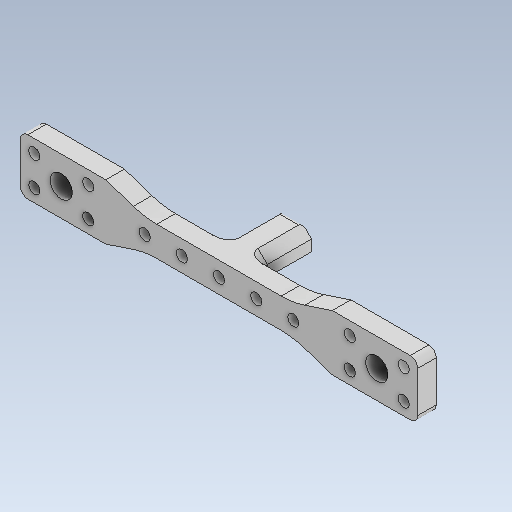
# Autodesk Inventor part: carbon_fiber_fixer_1
Saved by Autodesk Inventor 2020 (Build 240168000, 168)
## iProperties
Created: 2019-09-06
Part Number: carbon_fiber_fixer_1
Material: Generic
Document SubType Name: Modeling
Designer: psrob
Density: 1 g/cm^3
Appearance: Default
Author: psrob
Autodesk Inventor part; units mm, degrees
ref_plane "YZ Plane" through (0, 0, 0) normal (1, 0, 0) x (0, 1, 0)
ref_plane "XZ Plane" through (0, 0, 0) normal (0, 1, 0) x (-1, 0, 0)
ref_plane "XY Plane" through (0, 0, 0) normal (0, 0, 1) x (1, 0, 0)
sketch "Sketch1" plane through (0, 0, 0) normal (0, 0, 1) x (1, 0, 0)
  circle A0 centre (-100.25, -3.5) radius 1.5 projected
  circle A1 centre (-100.25, -11.5) radius 1.5 projected
  line L0 (-104, 0) -> (-96.5, 0) projected
  line L1 (-104, 0) -> (-104, -15) projected
  line L2 (-96.5, -15) -> (-104, -15) projected
  line L3 (-96.5, 0) -> (-96.5, -15) projected
  circle A2 centre (-85.75, -3.5) radius 1.5 projected
  circle A3 centre (-85.75, -11.5) radius 1.5 projected
  line L4 (-90.5, 0) -> (-81, 0) projected
  line L5 (-90.5, 0) -> (-90.5, -15) projected
  line L6 (-81, -15) -> (-90.5, -15) projected
  line L7 (-81, 0) -> (-81, -15) projected
  circle A4 centre (-15.25, -11.5) radius 1.5 projected
  circle A5 centre (-15.25, -3.5) radius 1.5 projected
  line L8 (-20, 0) -> (-10.5, 0) projected
  line L9 (-20, 0) -> (-20, -15) projected
  line L10 (-10.5, -15) -> (-20, -15) projected
  line L11 (-10.5, 0) -> (-10.5, -15) projected
  circle A6 centre (-0.75, -3.5) radius 1.5 projected
  circle A7 centre (-0.75, -11.5) radius 1.5 projected
  line L12 (-4.5, 0) -> (3, 0) projected
  line L13 (-4.5, 0) -> (-4.5, -15) projected
  line L14 (3, -15) -> (-4.5, -15) projected
  line L15 (3, 0) -> (3, -15) projected
  line L16 (-104, -15) -> (3, -15)
  line L17 (3, -15) -> (3, 0)
  line L18 (3, 0) -> (-104, 0)
  line L19 (-104, 0) -> (-104, -15)
  line L20 (-50.5, -15) -> (-50.5, 0)
  line L21 (-70.5, -11.5) -> (-70.5, -3.5)
  line L22 (-70.5, -3.5) -> (-30.5, -3.5)
  line L23 (-30.5, -3.5) -> (-30.5, -11.5)
  line L24 (-30.5, -11.5) -> (-70.5, -11.5)
  line L25 (-70.5, -11.5) -> (-30.5, -3.5) construction
  line L26 (-70.5, -3.5) -> (-30.5, -11.5) construction
  line L27 (-70.5, -3.5) -> (-81, 0)
  line L28 (-30.5, -3.5) -> (-20, 0)
  line L29 (-30.5, -11.5) -> (-20, -15)
  line L30 (-70.5, -11.5) -> (-81, -15)
  point P0 (0, 0)
  point P1 (-50.5, -7.5)
  dimension "d0" = 8
  dimension "d1" = 40
  constraints: 30 end point, 6 parallel, 5 midpoint, 2 perpendicular, 1 horizontal
  measures "d0" distance of L21.start L21.end
  measures "d1" distance of L21.end L22.end
extrude "Extrusion1" add sketch "Sketch1" along normal blind 5 contours L0 L3 L2 L1 | L18 L5 L16 L3 | L4 L7 L6 L5 | L27 L21 L30 L7 | L22 L20 L24 L21 | L8 L11 L10 L9 | L9 L29 L23 L28 | L22 L23 L24 L20 | L18 L13 L16 L11 | L12 L15 L14 L13
sketch "Sketch2" plane through (0, 0, 5) normal (0, 0, 1) x (1, 0, 0)
  line L0 (-81, 0) -> (-104, 0) projected
  line L1 (-104, 0) -> (-104, -15) projected
  line L2 (-104, -15) -> (-81, -15) projected
  line L3 (-81, -15) -> (-70.5, -11.5) projected
  line L4 (-70.5, -11.5) -> (-30.5, -11.5) projected
  line L5 (-30.5, -11.5) -> (-20, -15) projected
  line L6 (-20, -15) -> (3, -15) projected
  line L7 (3, -15) -> (3, 0) projected
  line L8 (3, 0) -> (-20, 0) projected
  line L9 (-20, 0) -> (-30.5, -3.5) projected
  line L10 (-30.5, -3.5) -> (-70.5, -3.5) projected
  line L11 (-70.5, -3.5) -> (-81, 0) projected
  circle A0 centre (-100.25, -3.5) radius 1.5 projected
  circle A1 centre (-100.25, -11.5) radius 1.5 projected
  circle A2 centre (-85.75, -3.5) radius 1.5 projected
  circle A3 centre (-85.75, -11.5) radius 1.5 projected
  circle A4 centre (-15.25, -11.5) radius 1.5 projected
  circle A5 centre (-15.25, -3.5) radius 1.5 projected
  circle A6 centre (-0.75, -3.5) radius 1.5 projected
  circle A7 centre (-0.75, -11.5) radius 1.5 projected
  line L12 (-70.5, -11.5) -> (-30.5, -11.5) projected
  line L13 (-50.5, -11.5) -> (-50.5, -3.5)
  line L14 (-30.5, -3.5) -> (-70.5, -3.5) projected
  line L15 (-50.5, -7.5) -> (-60.5, -7.5)
  line L16 (-60.5, -7.5) -> (-70.5, -7.5)
  line L17 (-50.5, -7.5) -> (-40.5, -7.5)
  line L18 (-40.5, -7.5) -> (-30.5, -7.5)
  circle A8 centre (-70.5, -7.5) radius 1.5
  circle A9 centre (-60.5, -7.5) radius 1.5
  circle A10 centre (-50.5, -7.5) radius 1.5
  circle A11 centre (-40.5, -7.5) radius 1.5
  circle A12 centre (-30.5, -7.5) radius 1.5
  point P0 (0, 0)
  dimension "d4" = 10
  dimension "d5" = 10
  dimension "d6" = 10
  dimension "d7" = 10
  dimension "d8" = 3
  dimension "d9" = 3
  dimension "d10" = 3
  dimension "d11" = 3
  dimension "d12" = 3
  constraints: 10 end point, 5 centre point, 5 coincident, 3 midpoint, 2 horizontal, 1 parallel, 1 point on line
  measures "d4" distance of L15.start L15.end
  measures "d5" distance of L15.end L16.end
  measures "d6" distance of L15.start L17.end
  measures "d7" distance of L17.end L18.end
  measures "d8" diameter of A8
  measures "d9" diameter of A9
  measures "d10" diameter of A10
  measures "d11" diameter of A11
  measures "d12" diameter of A12
extrude "Extrusion2" cut sketch "Sketch2" against normal blind 5 contours A10 L17 L13 | L13 L15 A10 | L17 A10 L13 | L13 A10 L15 | A9 L16 L15 | L15 L16 A9 | A11 L18 L17 | L17 L18 A11 | A8 | A12
fillet "Fillet1" radius 2 4 edges at (-104, 0, 2.5) (-104, -15, 2.5) (3, -15, 2.5) (3, 0, 2.5)
sketch "Sketch3" plane through (0, 0, 5) normal (0, 0, 1) x (1, 0, 0)
  arc A0 (3, -2) -> (1, 0) centre (1, -2) ccw projected
  line L0 (1, 0) -> (-20, 0) projected
  line L1 (-20, 0) -> (-30.5, -3.5) projected
  line L2 (-30.5, -3.5) -> (-70.5, -3.5) projected
  line L3 (-70.5, -3.5) -> (-81, 0) projected
  line L4 (-81, 0) -> (-102, 0) projected
  arc A1 (-102, 0) -> (-104, -2) centre (-102, -2) ccw projected
  line L5 (-104, -2) -> (-104, -13) projected
  arc A2 (-104, -13) -> (-102, -15) centre (-102, -13) ccw projected
  line L6 (-102, -15) -> (-81, -15) projected
  line L7 (-81, -15) -> (-70.5, -11.5) projected
  line L8 (-70.5, -11.5) -> (-30.5, -11.5) projected
  line L9 (-30.5, -11.5) -> (-20, -15) projected
  line L10 (-20, -15) -> (1, -15) projected
  arc A3 (1, -15) -> (3, -13) centre (1, -13) ccw projected
  line L11 (3, -13) -> (3, -2) projected
  circle A4 centre (-50.5, -7.5) radius 1.5 projected
  circle A5 centre (-40.5, -7.5) radius 1.5 projected
  circle A6 centre (-60.5, -7.5) radius 1.5 projected
  circle A7 centre (-30.5, -7.5) radius 1.5 projected
  circle A8 centre (-70.5, -7.5) radius 1.5 projected
  circle A9 centre (-100.25, -3.5) radius 1.5 projected
  circle A10 centre (-100.25, -11.5) radius 1.5 projected
  circle A11 centre (-85.75, -3.5) radius 1.5 projected
  circle A12 centre (-85.75, -11.5) radius 1.5 projected
  circle A13 centre (-15.25, -11.5) radius 1.5 projected
  circle A14 centre (-15.25, -3.5) radius 1.5 projected
  circle A15 centre (-0.75, -3.5) radius 1.5 projected
  circle A16 centre (-0.75, -11.5) radius 1.5 projected
  line L12 (-55.5, -11.5) -> (-55.5, -3.5)
  line L13 (-55.5, -3.5) -> (-45.5, -3.5)
  line L14 (-45.5, -3.5) -> (-45.5, -11.5)
  line L15 (-45.5, -11.5) -> (-55.5, -11.5)
  circle A17 centre (-50.5, -7.5) radius 1.5 projected
  line L16 (-55.5, -11.5) -> (-45.5, -3.5) construction
  line L17 (-55.5, -3.5) -> (-45.5, -11.5) construction
  point P0 (0, 0)
  dimension "d16" = 8
  dimension "d17" = 10
  constraints: 12 end point, 2 midpoint, 2 parallel, 1 perpendicular
  measures "d16" distance of L12.start L12.end
  measures "d17" distance of L12.end L13.end
ref_plane "Work Plane1" through (-77, -15, -14.9044) normal (0, 0, 1) x (1, 0, 0)
extrude "Extrusion3" add sketch "Sketch3" against normal up to surface (19.9044 mm away) contours L14 L8 L12 L2
chamfer "Chamfer1" distance 2.5 angle 45 4 edges at (-45.5, -3.5, -7.4522) (-55.5, -3.5, -7.4522) (-45.5, -11.5, -7.4522) (-55.5, -11.5, -7.4522)
fillet "Fillet2" radius 3 6 edges at (-54.25, -10.25, 0) (-55.5, -7.5, 0) (-54.25, -4.75, 0) (-46.75, -10.25, 0) (-45.5, -7.5, 0) (-46.75, -4.75, 0)
fillet "Fillet3" radius 1 1 edges at (-50.5, -3.5, -14.9044)
fillet "Fillet4" radius 20 4 edges at (-70.5, -3.5, 2.5) (-30.5, -3.5, 2.5) (-70.5, -11.5, 2.5) (-30.5, -11.5, 2.5)
sketch "Sketch4" plane through (0, 0, 5) normal (0, 0, 1) x (1, 0, 0)
  circle A0 centre (-0.75, -11.5) radius 1.5 projected
  circle A1 centre (-0.75, -3.5) radius 1.5 projected
  circle A2 centre (-15.25, -3.5) radius 1.5 projected
  circle A3 centre (-15.25, -11.5) radius 1.5 projected
  circle A4 centre (-30.5, -7.5) radius 1.5 projected
  circle A5 centre (-40.5, -7.5) radius 1.5 projected
  circle A6 centre (-50.5, -7.5) radius 1.5 projected
  line L0 (-33.7456, -3.5) -> (-67.2544, -3.5) projected
  arc A7 (-73.579, -2.4737) -> (-67.2544, -3.5) centre (-67.2544, 16.5) ccw projected
  line L1 (-73.579, -2.4737) -> (-81, 0) projected
  line L2 (-81, 0) -> (-102, 0) projected
  arc A8 (-102, 0) -> (-104, -2) centre (-102, -2) ccw projected
  line L3 (-104, -2) -> (-104, -13) projected
  arc A9 (-104, -13) -> (-102, -15) centre (-102, -13) ccw projected
  line L4 (-102, -15) -> (-81, -15) projected
  line L5 (-81, -15) -> (-73.579, -12.5263) projected
  arc A10 (-67.2544, -11.5) -> (-73.579, -12.5263) centre (-67.2544, -31.5) ccw projected
  line L6 (-67.2544, -11.5) -> (-33.7456, -11.5) projected
  arc A11 (-27.421, -12.5263) -> (-33.7456, -11.5) centre (-33.7456, -31.5) ccw projected
  line L7 (-27.421, -12.5263) -> (-20, -15) projected
  line L8 (-20, -15) -> (1, -15) projected
  arc A12 (1, -15) -> (3, -13) centre (1, -13) ccw projected
  line L9 (3, -13) -> (3, -2) projected
  arc A13 (3, -2) -> (1, 0) centre (1, -2) ccw projected
  line L10 (1, 0) -> (-20, 0) projected
  line L11 (-20, 0) -> (-27.421, -2.4737) projected
  arc A14 (-33.7456, -3.5) -> (-27.421, -2.4737) centre (-33.7456, 16.5) ccw projected
  circle A15 centre (-60.5, -7.5) radius 1.5 projected
  circle A16 centre (-70.5, -7.5) radius 1.5 projected
  circle A17 centre (-100.25, -3.5) radius 1.5 projected
  circle A18 centre (-100.25, -11.5) radius 1.5 projected
  circle A19 centre (-85.75, -3.5) radius 1.5 projected
  circle A20 centre (-85.75, -11.5) radius 1.5 projected
  line L12 (-100.25, -3.5) -> (-85.75, -11.5)
  circle A21 centre (-85.75, -3.5) radius 1.5 projected
  line L13 (-85.75, -11.5) -> (-85.75, -3.5)
  circle A22 centre (-100.25, -11.5) radius 1.5 projected
  line L14 (-85.75, -3.5) -> (-100.25, -11.5)
  circle A23 centre (-15.25, -11.5) radius 1.5 projected
  line L15 (-0.75, -3.5) -> (-15.25, -11.5)
  line L16 (-15.25, -11.5) -> (-15.25, -3.5)
  circle A24 centre (-0.75, -11.5) radius 1.5 projected
  line L17 (-15.25, -3.5) -> (-0.75, -11.5)
  circle A25 centre (-93, -7.5) radius 3
  circle A26 centre (-8, -7.5) radius 3
  point P0 (0, 0)
  dimension "d26" = 6
  dimension "d27" = 6
  constraints: 12 end point, 2 centre point, 2 midpoint, 2 vertical
  measures "d26" diameter of A25
  measures "d27" diameter of A26
extrude "Extrusion4" cut sketch "Sketch4" against normal blind 5 contours A26 L15 L17 | L17 L15 A26 | L17 A26 L15 | L15 A26 L17 | A25 L12 L14 | L14 L12 A25 | L14 A25 L12 | L12 A25 L14
body "Solid1"
